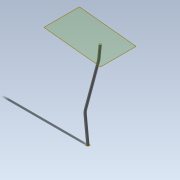
# Autodesk Inventor part: NoseBentBar
Saved by Autodesk Inventor 2020 (Build 240168000, 168)
## iProperties
Created: 2021-07-09
Part Number: NoseBentBar
Material: Generic
Document SubType Name: Modeling
Designer: Val
Density: 1 g/cm^3
Appearance: Default
Author: Val
Autodesk Inventor part; units mm, degrees
ref_plane "YZ Plane" through (0, 0, 0) normal (1, 0, 0) x (0, 1, 0)
ref_plane "XZ Plane" through (0, 0, 0) normal (0, 1, 0) x (-1, 0, 0)
ref_plane "XY Plane" through (0, 0, 0) normal (0, 0, 1) x (1, 0, 0)
sketch "BaseProfile" plane through (0, 0, 0) normal (0, 0, 1) x (1, 0, 0)
  line L0 (-5.4941, -149.1667) -> (-9.4725, -148.752) projected
  line L1 (-9.5036, -165.3253) -> (-31.5674, -247.9528)
  line L2 (-16.8134, -161.3043) -> (-40.3905, -249.5992) construction
  line L3 (-15.5803, -135.6093) -> (-16.8134, -161.3043) construction
  line L4 (-8.9879, -163.3939) -> (-16.8134, -161.3043) construction
  line L5 (-6.3546, -138.1308) -> (-8.7806, -161.4057)
  line L6 (-32.284, -257.199) -> (-27.7247, -299.9552)
  arc A0 (-9.5036, -165.3253) -> (-8.7806, -161.4057) centre (-34.0438, -158.7724) ccw
  arc A1 (-31.5674, -247.9528) -> (-32.284, -257.199) centre (-7.0272, -254.5057) ccw
  point P0 (0, 0)
  point P1 (-32.7841, -252.5093)
  point P2 (-7.4833, -148.9594)
  dimension "d1" = 25.4
  dimension "d3" = 47.7149
  dimension "d7" = 25.4
  dimension "d8" = 171
  constraints: 10 end point, 5 point on line, 4 point on circle, 4 tangent, 2 centre point, 2 perpendicular, 1 equal radius, 1 midpoint, 1 parallel
  measures "d1" distance of L5.start L4.start
  measures "d3" distance of point (-32.784, -252.509) L6.end
  measures "d7" radius of A0
  measures "d8" angle of L1 L5
ref_plane "SweepPlane" through (-6.3546, -138.1308, 0) normal (-0.1037, -0.9946, 0) x (0, 0, 1)
ref_plane "Work Plane1" through (-7.4833, -148.9594, -12.7182) normal (-0.1037, -0.9946, 0) x (0, 0, 1)
sketch "Sketch2" plane through (-6.3546, -138.1308, 0) normal (-0.1037, -0.9946, 0) x (0, 0, 1)
  circle A0 centre (0, 0) radius 2
  point P0 (0, 8)
  dimension "d4" = 4
  constraints: 1 centre point, 1 coincident
  measures "d4" diameter of A0
sweep "SweepFeature" add profiles "Sketch2" path "BaseProfile" path curves L5 A0 L1 A1 L6
ref_plane "EndSweepPlane" through (-27.7247, -299.9552, 0) normal (0.106, -0.9944, 0) x (0.9944, 0.106, 0)
body "Solid1"
